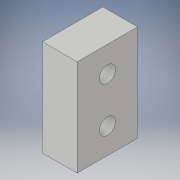
# Autodesk Inventor part: SliderBlock
Saved by Autodesk Inventor 2019 (Build 230136000, 136)
## iProperties
Created: 2019-09-28
Part Number: SliderBlock
Material: Generic
Document SubType Name: Modeling
Designer: james
Density: 1 g/cm^3
Appearance: Default
Mass: 1.5506 g
Surface Area: 10.2449 cm^2
Volume: 1.5506 cm^3
Author: james
Autodesk Inventor part; units mm, degrees
ref_plane "YZ Plane" through (0, 0, 0) normal (1, 0, 0) x (0, 1, 0)
ref_plane "XZ Plane" through (0, 0, 0) normal (0, 1, 0) x (-1, 0, 0)
ref_plane "XY Plane" through (0, 0, 0) normal (0, 0, 1) x (1, 0, 0)
sketch "Sketch1" plane through (0, 0, 0) normal (1, 0, 0) x (0, 1, 0)
  line L0 (12.0622, 21.4347) -> (-6.9878, 21.4347)
  line L1 (-6.9878, 21.4347) -> (-6.9878, 8.7347)
  line L2 (-6.9878, 8.7347) -> (12.0622, 8.7347)
  line L3 (12.0622, 8.7347) -> (12.0622, 21.4347)
  point P0 (0, 0)
  dimension "d0" = 12.7
  dimension "d1" = 19.05
  constraints: 8 end point, 2 parallel, 1 horizontal, 1 perpendicular
  measures "d0" distance of L2.end L0.start
  measures "d1" distance of L0.start L0.end
extrude "Extrusion1" add sketch "Sketch1" along normal blind 6.858
sketch "Sketch2" plane through (6.858, 0, 0) normal (1, 0, 0) x (0, 0, -1)
  line L0 (-8.7347, -6.9878) -> (-8.7347, 12.0622) projected
  line L1 (-8.7347, 12.0622) -> (-21.4347, 12.0622) projected
  point P0 (0, 0)
  point P1 (-15.0847, 6.9822)
  point P2 (-15.0847, -1.9078)
  dimension "d4" = 6.35
  dimension "d5" = 6.35
  dimension "d6" = 13.97
  dimension "d7" = 5.08
  measures "d4" distance from line of L0 point (-15.085, 6.982)
  measures "d5" distance from line of L0 point (-15.085, -1.908)
  measures "d6" distance from line of L1 point (-15.085, -1.908)
  measures "d7" distance from line of L1 point (-15.085, 6.982)
hole "Hole1" at (6.858, 6.9822, 15.0847) at (6.858, -1.9078, 15.0847) direction (-1, 0, 0) diameter 3.175 end through all
sketch "Sketch3" plane through (6.858, 0, 0) normal (1, 0, 0) x (0, 0, -1)
  line L0 (-23.9685, 13.1299) -> (-21.0537, 13.1299)
  line L1 (-21.0537, 13.1299) -> (-21.0537, -8.0318)
  line L2 (-21.0537, -8.0318) -> (-23.9685, -8.0318)
  line L3 (-23.9685, -8.0318) -> (-23.9685, 13.1299)
  line L4 (-7.9023, 13.3864) -> (-9.1157, 13.3864)
  line L5 (-9.1157, 13.3864) -> (-9.1157, -8.3525)
  line L6 (-9.1157, -8.3525) -> (-7.9023, -8.3525)
  line L7 (-7.9023, -8.3525) -> (-7.9023, 13.3864)
  line L8 (-21.4347, 12.0622) -> (-21.4347, -6.9878) projected
  line L9 (-8.7347, -6.9878) -> (-8.7347, 12.0622) projected
  point P0 (0, 0)
  dimension "d15" = 0.381
  dimension "d16" = 0.381
  constraints: 16 end point, 4 parallel, 2 horizontal, 2 perpendicular
  measures "d15" distance between parallel lines of L8 L1
  measures "d16" distance between parallel lines of L9 L5
extrude "Extrusion2" cut sketch "Sketch3" against normal blind 25.4
body "Solid1"
